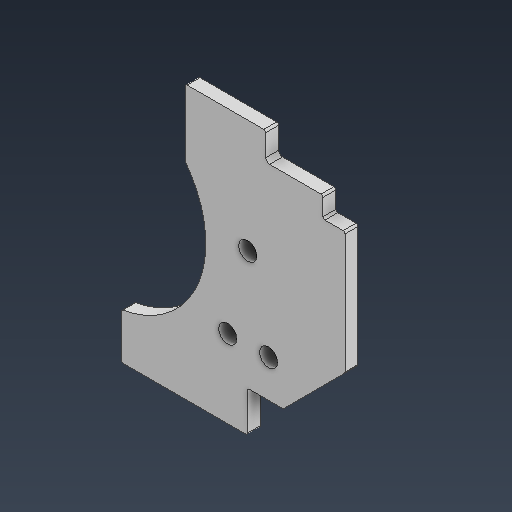
# Autodesk Inventor part: mount_carriage_bottom
Saved by Autodesk Inventor 2021 (Build 250183000, 183)
## iProperties
Created: 2020-12-29
Part Number: mount_carriage_bottom
Material: Generic
Document SubType Name: Modeling
Designer: Tomasz
Density: 1 g/cm^3
Appearance: Default
Author: Tomasz
Autodesk Inventor part; units mm, degrees
ref_plane "YZ Plane" through (0, 0, 0) normal (1, 0, 0) x (0, 1, 0)
ref_plane "XZ Plane" through (0, 0, 0) normal (0, 1, 0) x (-1, 0, 0)
ref_plane "XY Plane" through (0, 0, 0) normal (0, 0, 1) x (1, 0, 0)
ref_plane "Work Plane1" through (-17.3538, -25.3153, -5.1) normal (0, 0, 1) x (1, 0, 0)
sketch "holes" plane through (0, 0, 0) normal (0, 0, 1) x (1, 0, 0)
  arc A0 (17.3538, 10.1647) -> (17.0538, 10.4647) centre (17.0538, 10.1647) ccw
  line L0 (17.0538, 10.4647) -> (14.2323, 10.4647)
  arc A1 (13.9323, 10.7647) -> (14.2323, 10.4647) centre (14.2323, 10.7647) ccw
  line L1 (13.9323, 10.7647) -> (13.9323, 13.3588)
  arc A2 (13.9323, 13.3588) -> (13.6323, 13.6588) centre (13.6323, 13.3588) ccw
  line L2 (13.6323, 13.6588) -> (5.6606, 13.6588)
  arc A3 (5.0636, 14.2558) -> (5.6606, 13.6588) centre (5.6606, 14.2558) ccw
  line L3 (5.0636, 14.2558) -> (5.0636, 17.6129)
  arc A4 (5.0636, 17.6129) -> (4.7636, 17.9129) centre (4.7636, 17.6129) ccw
  line L4 (4.7636, 17.9129) -> (-1.9383, 17.9129)
  arc A5 (-2.2383, 18.2129) -> (-1.9383, 17.9129) centre (-1.9383, 18.2129) ccw
  line L5 (-2.2383, 18.2129) -> (-2.2383, 18.3742)
  arc A6 (-2.2383, 18.3742) -> (-2.5383, 18.6742) centre (-2.5383, 18.3742) ccw
  line L6 (-2.5383, 18.6742) -> (-3.5364, 18.6742)
  arc A7 (-3.8364, 18.9742) -> (-3.5364, 18.6742) centre (-3.5364, 18.9742) ccw
  line L7 (-3.8364, 18.9742) -> (-3.8364, 19.9671)
  arc A8 (-3.8364, 19.9671) -> (-4.1364, 20.2671) centre (-4.1364, 19.9671) ccw
  line L8 (-4.1364, 20.2671) -> (-5.1364, 20.2671)
  arc A9 (-5.4364, 20.5671) -> (-5.1364, 20.2671) centre (-5.1364, 20.5671) ccw
  line L9 (-5.4364, 20.5671) -> (-5.4364, 24.1018)
  arc A10 (-5.4364, 24.1018) -> (-5.7364, 24.4018) centre (-5.7364, 24.1018) ccw
  line L10 (-5.7364, 24.4018) -> (-7.1364, 24.4018)
  arc A11 (-7.1364, 24.4018) -> (-7.4364, 24.1018) centre (-7.1364, 24.1018) ccw
  line L11 (-7.4364, 24.1018) -> (-7.4364, 7.6483)
  arc A12 (-7.4364, 7.6483) -> (-7.3759, 7.4677) centre (-7.1364, 7.6483) ccw
  arc A13 (-17.115, -17.2892) -> (-7.3759, 7.4677) centre (-19.8297, -1.9272) ccw
  arc A14 (-17.115, -17.2892) -> (-17.3538, -17.5116) centre (-17.0628, -17.5846) ccw
  line L12 (-17.3538, -17.5116) -> (-17.3538, -24.1018)
  arc A15 (-17.3538, -24.1018) -> (-17.0538, -24.4018) centre (-17.0538, -24.1018) ccw
  line L13 (-17.0538, -24.4018) -> (1.9557, -24.4018)
  arc A16 (1.9557, -24.4018) -> (2.2557, -24.1018) centre (1.9557, -24.1018) ccw
  line L14 (2.2557, -24.1018) -> (2.2557, -18.3961)
  arc A17 (2.5557, -18.0961) -> (2.2557, -18.3961) centre (2.5557, -18.3961) ccw
  line L15 (2.5557, -18.0961) -> (7.6549, -18.0961)
  arc A18 (7.6549, -18.0961) -> (7.8673, -18.008) centre (7.6549, -17.7961) ccw
  line L16 (7.8673, -18.008) -> (17.2662, -8.5819)
  arc A19 (17.2662, -8.5819) -> (17.3538, -8.3701) centre (17.0538, -8.3701) ccw
  line L17 (17.3538, -8.3701) -> (17.3538, 10.1647)
  arc A20 (1.196, -8.6701) -> (1.3547, -8.6247) centre (1.196, -8.3701) ccw
  line L18 (1.3547, -8.6247) -> (2.0283, -8.2049)
  arc A21 (2.3456, -8.2049) -> (2.0283, -8.2049) centre (2.187, -8.4595) ccw
  line L19 (2.3456, -8.2049) -> (3.0192, -8.6247)
  arc A22 (3.0192, -8.6247) -> (3.1779, -8.6701) centre (3.1779, -8.3701) ccw
  line L20 (3.1779, -8.6701) -> (7.8974, -8.6701)
  arc A23 (8.8974, -9.6701) -> (7.8974, -8.6701) centre (7.8974, -9.6701) ccw
  line L21 (8.8974, -9.6701) -> (8.8974, -14.0729)
  arc A24 (8.8069, -14.2875) -> (8.8974, -14.0729) centre (8.5974, -14.0729) ccw
  line L22 (8.8069, -14.2875) -> (7.1705, -15.8848)
  arc A25 (6.9609, -15.9701) -> (7.1705, -15.8848) centre (6.9609, -15.6701) ccw
  line L23 (6.9609, -15.9701) -> (-2.2459, -15.9701)
  arc A26 (-2.4611, -15.8791) -> (-2.2459, -15.9701) centre (-2.2459, -15.6701) ccw
  line L24 (-2.4611, -15.8791) -> (-4.1564, -14.1338)
  arc A27 (-4.2412, -13.9247) -> (-4.1564, -14.1338) centre (-3.9412, -13.9247) ccw
  line L25 (-4.2412, -13.9247) -> (-4.2412, -9.6701)
  arc A28 (-3.2412, -8.6701) -> (-4.2412, -9.6701) centre (-3.2412, -9.6701) ccw
  line L26 (-3.2412, -8.6701) -> (1.196, -8.6701)
  arc A29 (4.2967, -2.4382) -> (3.9967, -2.1382) centre (3.9967, -2.4382) ccw
  line L27 (3.9967, -2.1382) -> (0.6538, -2.1382)
  arc A30 (0.6538, -2.1382) -> (0.3538, -2.4382) centre (0.6538, -2.4382) ccw
  line L28 (0.3538, -2.4382) -> (0.3538, -6.5942)
  arc A31 (0.0538, -6.8942) -> (0.3538, -6.5942) centre (0.0538, -6.5942) ccw
  line L29 (0.0538, -6.8942) -> (-2.1438, -6.8942)
  arc A32 (-2.4438, -6.5942) -> (-2.1438, -6.8942) centre (-2.1438, -6.5942) ccw
  line L30 (-2.4438, -6.5942) -> (-2.4438, -3.9753)
  arc A33 (-2.4438, -3.9753) -> (-2.1438, -3.6753) centre (-2.4438, -3.6753) ccw
  line L31 (-2.1438, -3.6753) -> (-2.1438, -0.4348)
  arc A34 (-2.1438, -0.4348) -> (-2.4438, -0.1348) centre (-2.4438, -0.4348) ccw
  line L32 (-2.4438, -0.1348) -> (-2.4438, 2.5284)
  arc A35 (-2.1438, 2.8284) -> (-2.4438, 2.5284) centre (-2.1438, 2.5284) ccw
  line L33 (-2.1438, 2.8284) -> (6.6827, 2.8284)
  arc A36 (6.9827, 2.5284) -> (6.6827, 2.8284) centre (6.6827, 2.5284) ccw
  line L34 (6.9827, 2.5284) -> (6.9827, -0.1348)
  arc A37 (6.9827, -0.1348) -> (6.6827, -0.4348) centre (6.9827, -0.4348) ccw
  line L35 (6.6827, -0.4348) -> (6.6827, -3.6753)
  arc A38 (6.6827, -3.6753) -> (6.9827, -3.9753) centre (6.9827, -3.6753) ccw
  line L36 (6.9827, -3.9753) -> (6.9827, -6.5942)
  arc A39 (6.6827, -6.8942) -> (6.9827, -6.5942) centre (6.6827, -6.5942) ccw
  line L37 (6.6827, -6.8942) -> (4.5967, -6.8942)
  arc A40 (4.2967, -6.5942) -> (4.5967, -6.8942) centre (4.5967, -6.5942) ccw
  line L38 (4.2967, -6.5942) -> (4.2967, -2.4382)
  circle A41 centre (2.2695, 0.3451) radius 1.4
  circle A42 centre (5.4974, -12.3201) radius 1.4
  circle A43 centre (-0.8412, -12.3201) radius 1.4
  line L39 (-7.1364, 17.9129) -> (4.7636, 17.9129)
  arc A44 (-7.1364, 17.9129) -> (-7.4364, 17.6129) centre (-7.1364, 17.6129) ccw
  line L40 (-7.4364, 7.6483) -> (-7.4364, 17.6129)
  point P0 (0, 0)
extrude "Extrusion1" add sketch "holes" against normal up to surface (5.1 mm away) contours A20 L18 A21 L19 A22 L20 A23 L21 A24 L22 A25 L23 A26 L24 A27 L25 A28 L26 | A29 L27 A30 L28 A31 L29 A32 L30 A33 L31 A34 L32 A35 L33 A36 L34 A37 L35 A38 L36 A39 L37 A40 L38
ref_plane "Work Plane2" through (280.5257, 0, 0) normal (0, 0, 1) x (1, 0, 0)
sketch "plate" plane through (0, 0, 0) normal (0, 0, 1) x (1, 0, 0)
  arc A0 (17.3538, 10.1647) -> (17.0538, 10.4647) centre (17.0538, 10.1647) ccw projected
  line L0 (17.0538, 10.4647) -> (14.2323, 10.4647) projected
  arc A1 (13.9323, 10.7647) -> (14.2323, 10.4647) centre (14.2323, 10.7647) ccw projected
  line L1 (13.9323, 10.7647) -> (13.9323, 13.3588) projected
  arc A2 (13.9323, 13.3588) -> (13.6323, 13.6588) centre (13.6323, 13.3588) ccw projected
  line L2 (13.6323, 13.6588) -> (5.6606, 13.6588) projected
  arc A3 (5.0636, 14.2558) -> (5.6606, 13.6588) centre (5.6606, 14.2558) ccw projected
  line L3 (5.0636, 14.2558) -> (5.0636, 17.6129) projected
  arc A4 (5.0636, 17.6129) -> (4.7636, 17.9129) centre (4.7636, 17.6129) ccw projected
  line L4 (4.7636, 17.9129) -> (-1.9383, 17.9129) projected
  arc A5 (-2.2383, 18.2129) -> (-1.9383, 17.9129) centre (-1.9383, 18.2129) ccw projected
  line L5 (-2.2383, 18.2129) -> (-2.2383, 18.3742) projected
  arc A6 (-2.2383, 18.3742) -> (-2.5383, 18.6742) centre (-2.5383, 18.3742) ccw projected
  line L6 (-2.5383, 18.6742) -> (-3.5364, 18.6742) projected
  arc A7 (-3.8364, 18.9742) -> (-3.5364, 18.6742) centre (-3.5364, 18.9742) ccw projected
  line L7 (-3.8364, 18.9742) -> (-3.8364, 19.9671) projected
  arc A8 (-3.8364, 19.9671) -> (-4.1364, 20.2671) centre (-4.1364, 19.9671) ccw projected
  line L8 (-4.1364, 20.2671) -> (-5.1364, 20.2671) projected
  arc A9 (-5.4364, 20.5671) -> (-5.1364, 20.2671) centre (-5.1364, 20.5671) ccw projected
  line L9 (-5.4364, 20.5671) -> (-5.4364, 24.1018) projected
  arc A10 (-5.4364, 24.1018) -> (-5.7364, 24.4018) centre (-5.7364, 24.1018) ccw projected
  line L10 (-5.7364, 24.4018) -> (-7.1364, 24.4018) projected
  arc A11 (-7.1364, 24.4018) -> (-7.4364, 24.1018) centre (-7.1364, 24.1018) ccw projected
  line L11 (-7.4364, 24.1018) -> (-7.4364, 7.6483) projected
  arc A12 (-7.4364, 7.6483) -> (-7.3759, 7.4677) centre (-7.1364, 7.6483) ccw projected
  arc A13 (-17.115, -17.2892) -> (-7.3759, 7.4677) centre (-19.8297, -1.9272) ccw projected
  arc A14 (-17.115, -17.2892) -> (-17.3538, -17.5116) centre (-17.0628, -17.5846) ccw projected
  line L12 (-17.3538, -17.5116) -> (-17.3538, -24.1018) projected
  arc A15 (-17.3538, -24.1018) -> (-17.0538, -24.4018) centre (-17.0538, -24.1018) ccw projected
  line L13 (-17.0538, -24.4018) -> (1.9557, -24.4018) projected
  arc A16 (1.9557, -24.4018) -> (2.2557, -24.1018) centre (1.9557, -24.1018) ccw projected
  line L14 (2.2557, -24.1018) -> (2.2557, -18.3961) projected
  arc A17 (2.5557, -18.0961) -> (2.2557, -18.3961) centre (2.5557, -18.3961) ccw projected
  line L15 (2.5557, -18.0961) -> (7.6549, -18.0961) projected
  arc A18 (7.6549, -18.0961) -> (7.8673, -18.008) centre (7.6549, -17.7961) ccw projected
  line L16 (7.8673, -18.008) -> (17.2662, -8.5819) projected
  arc A19 (17.2662, -8.5819) -> (17.3538, -8.3701) centre (17.0538, -8.3701) ccw projected
  line L17 (17.3538, -8.3701) -> (17.3538, 10.1647) projected
  arc A20 (1.196, -8.6701) -> (1.3547, -8.6247) centre (1.196, -8.3701) ccw projected
  line L18 (1.3547, -8.6247) -> (2.0283, -8.2049) projected
  arc A21 (2.3456, -8.2049) -> (2.0283, -8.2049) centre (2.187, -8.4595) ccw projected
  line L19 (2.3456, -8.2049) -> (3.0192, -8.6247) projected
  arc A22 (3.0192, -8.6247) -> (3.1779, -8.6701) centre (3.1779, -8.3701) ccw projected
  line L20 (3.1779, -8.6701) -> (7.8974, -8.6701) projected
  arc A23 (8.8974, -9.6701) -> (7.8974, -8.6701) centre (7.8974, -9.6701) ccw projected
  line L21 (8.8974, -9.6701) -> (8.8974, -14.0729) projected
  arc A24 (8.8069, -14.2875) -> (8.8974, -14.0729) centre (8.5974, -14.0729) ccw projected
  line L22 (8.8069, -14.2875) -> (7.1705, -15.8848) projected
  arc A25 (6.9609, -15.9701) -> (7.1705, -15.8848) centre (6.9609, -15.6701) ccw projected
  line L23 (6.9609, -15.9701) -> (-2.2459, -15.9701) projected
  arc A26 (-2.4611, -15.8791) -> (-2.2459, -15.9701) centre (-2.2459, -15.6701) ccw projected
  line L24 (-2.4611, -15.8791) -> (-4.1564, -14.1338) projected
  arc A27 (-4.2412, -13.9247) -> (-4.1564, -14.1338) centre (-3.9412, -13.9247) ccw projected
  line L25 (-4.2412, -13.9247) -> (-4.2412, -9.6701) projected
  arc A28 (-3.2412, -8.6701) -> (-4.2412, -9.6701) centre (-3.2412, -9.6701) ccw projected
  line L26 (-3.2412, -8.6701) -> (1.196, -8.6701) projected
  arc A29 (4.2967, -2.4382) -> (3.9967, -2.1382) centre (3.9967, -2.4382) ccw projected
  line L27 (3.9967, -2.1382) -> (0.6538, -2.1382) projected
  arc A30 (0.6538, -2.1382) -> (0.3538, -2.4382) centre (0.6538, -2.4382) ccw projected
  line L28 (0.3538, -2.4382) -> (0.3538, -6.5942) projected
  arc A31 (0.0538, -6.8942) -> (0.3538, -6.5942) centre (0.0538, -6.5942) ccw projected
  line L29 (0.0538, -6.8942) -> (-2.1438, -6.8942) projected
  arc A32 (-2.4438, -6.5942) -> (-2.1438, -6.8942) centre (-2.1438, -6.5942) ccw projected
  line L30 (-2.4438, -6.5942) -> (-2.4438, -3.9753) projected
  arc A33 (-2.4438, -3.9753) -> (-2.1438, -3.6753) centre (-2.4438, -3.6753) ccw projected
  line L31 (-2.1438, -3.6753) -> (-2.1438, -0.4348) projected
  arc A34 (-2.1438, -0.4348) -> (-2.4438, -0.1348) centre (-2.4438, -0.4348) ccw projected
  line L32 (-2.4438, -0.1348) -> (-2.4438, 2.5284) projected
  arc A35 (-2.1438, 2.8284) -> (-2.4438, 2.5284) centre (-2.1438, 2.5284) ccw projected
  line L33 (-2.1438, 2.8284) -> (6.6827, 2.8284) projected
  arc A36 (6.9827, 2.5284) -> (6.6827, 2.8284) centre (6.6827, 2.5284) ccw projected
  line L34 (6.9827, 2.5284) -> (6.9827, -0.1348) projected
  arc A37 (6.9827, -0.1348) -> (6.6827, -0.4348) centre (6.9827, -0.4348) ccw projected
  line L35 (6.6827, -0.4348) -> (6.6827, -3.6753) projected
  arc A38 (6.6827, -3.6753) -> (6.9827, -3.9753) centre (6.9827, -3.6753) ccw projected
  line L36 (6.9827, -3.9753) -> (6.9827, -6.5942) projected
  arc A39 (6.6827, -6.8942) -> (6.9827, -6.5942) centre (6.6827, -6.5942) ccw projected
  line L37 (6.6827, -6.8942) -> (4.5967, -6.8942) projected
  arc A40 (4.2967, -6.5942) -> (4.5967, -6.8942) centre (4.5967, -6.5942) ccw projected
  line L38 (4.2967, -6.5942) -> (4.2967, -2.4382) projected
  arc A41 (-7.1364, 17.9129) -> (-7.4364, 17.6129) centre (-7.1364, 17.6129) ccw projected
  line L39 (-7.1364, 17.9129) -> (4.7636, 17.9129) projected
  circle A42 centre (2.2695, 0.3451) radius 1.4 projected
  circle A43 centre (5.4974, -12.3201) radius 1.4 projected
  circle A44 centre (-0.8412, -12.3201) radius 1.4 projected
  point P0 (0, 0)
extrude "Extrusion2" add sketch "plate" along normal blind 2 contours L17 A19 L16 A18 L15 A17 L14 A16 L13 A15 L12 A14 A13 A12 L11 A41 L39 L4 A4 L3 A3 L2 A2 L1 A1 L0 A0 | A20 L18 A21 L19 A22 L20 A23 L21 A24 L22 A25 L23 A26 L24 A27 L25 A28 L26 | A29 L27 A30 L28 A31 L29 A32 L30 A33 L31 A34 L32 A35 L33 A36 L34 A37 L35 A38 L36 A39 L37 A40 L38
body "Solid1"
